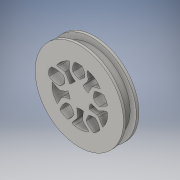
# Autodesk Inventor part: Desgin on wheel
Saved by Autodesk Inventor 2016 (Build 200138000, 138)
## iProperties
Created: 2017-09-08
Part Number: Desgin on wheel
Material: Generic
Document SubType Name: Modeling
Designer: student
Density: 1 g/cm^3
Appearance: Default
Author: student
Autodesk Inventor part; units mm, degrees
ref_plane "YZ Plane" through (0, 0, 0) normal (1, 0, 0) x (0, 1, 0)
ref_plane "XZ Plane" through (0, 0, 0) normal (0, 1, 0) x (-1, 0, 0)
ref_plane "XY Plane" through (0, 0, 0) normal (0, 0, 1) x (1, 0, 0)
sketch "Sketch1" plane through (0, 0, 0) normal (0, 0, 1) x (1, 0, 0)
  circle A0 centre (0, 0) radius 4.826
  dimension "d0" = 9.652
  constraints: 1 centre point, 1 coincident
  measures "d0" diameter of A0
extrude "Extrusion1" add sketch "Sketch1" along normal blind 3.048
sketch "Sketch2" plane through (0, 0, 3.048) normal (0, 0, 1) x (1, 0, 0)
  circle A0 centre (0, 0) radius 22.86
  dimension "d3" = 45.72
  constraints: 1 centre point, 1 coincident
  measures "d3" diameter of A0
extrude "Extrusion2" add sketch "Sketch2" along normal blind 1.397
sketch "Sketch4" plane through (0, 0, 4.445) normal (0, 0, 1) x (1, 0, 0)
  circle A0 centre (0, 0) radius 19.685
  dimension "d6" = 39.37
  constraints: 1 centre point, 1 coincident
  measures "d6" diameter of A0
extrude "Extrusion3" add sketch "Sketch4" along normal blind 5.334
sketch "Sketch6" plane through (0, 0, 9.779) normal (0, 0, 1) x (1, 0, 0)
  circle A0 centre (0, 0) radius 4.826 projected
  circle A1 centre (0, 0) radius 22.86
  constraints: 1 centre point, 1 coincident
extrude "Extrusion4" add sketch "Sketch6" along normal blind 1.27 contours A0 | A1
sketch "Sketch9" plane through (0, 0, 0) normal (0, 0, -1) x (-1, 0, 0)
  line L0 (2.3876, -2.514) -> (2.3876, 2.514)
  line L1 (-2.3876, 2.514) -> (-2.3876, -2.514)
  line L2 (-1.2735, -3.2247) -> (1.2735, 3.2247) construction
  line L3 (1.2735, -3.2247) -> (-1.2735, 3.2247) construction
  arc A0 (-2.3876, -2.514) -> (2.3876, -2.514) centre (0, 0) ccw
  arc A1 (2.3876, 2.514) -> (-2.3876, 2.514) centre (0, 0) ccw
  constraints: 8 end point, 8 point on circle, 2 centre point, 2 midpoint, 1 coincident, 1 parallel
extrude "Extrusion6" cut sketch "Sketch9" against normal blind 5.5118
sketch "Sketch10" plane through (0, 0, 3.048) normal (0, 0, -1) x (-1, 0, 0)
  arc A0 (6.0888, 12.8089) -> (4.9517, 12.8553) centre (5.4971, 12.2636) ccw
  arc A1 (11.5392, 8.311) -> (6.0888, 12.8089) centre (0.4834, 0.4651) ccw
  arc A2 (11.0546, 7.7734) -> (11.5392, 8.311) centre (11.2368, 8.0964) ccw
  arc A3 (11.0546, 7.7734) -> (7.4347, 7.1004) centre (11.1442, -2.7813) ccw
  circle A4 centre (0, 0) radius 22.86 projected
  arc A5 (5.2433, 9.0758) -> (4.9517, 12.8553) centre (-169.1009, -2.4734) ccw
  arc A6 (2.0036, 5.6242) -> (5.2433, 9.0758) centre (-1.766, 12.4088) ccw
  arc A7 (2.0036, 5.6242) -> (4.9517, 3.0409) centre (11.897, 13.941) ccw
  arc A8 (7.4347, 7.1004) -> (4.9517, 3.0409) centre (16.2062, -1.0536) ccw
  arc A9 (11.2368, -8.9724) -> (14.0004, -0.5744) centre (4.7112, -2.1713) ccw
  arc A10 (9.1497, -5.1175) -> (11.2368, -8.9724) centre (208.9836, 100.5866) ccw
  arc A11 (9.1497, -5.1175) -> (4.7112, -3.7562) centre (4.4946, -12.3784) ccw
  arc A12 (5.8832, -0.5744) -> (4.7112, -3.7562) centre (18.9185, -7.1827) ccw
  arc A13 (5.8832, -0.5744) -> (9.9506, -2.3296) centre (12.8849, 10.061) ccw
  arc A14 (9.9506, -2.3296) -> (14.0004, -0.5744) centre (5.7085, 13.0084) ccw
  arc A15 (9.9506, -11.266) -> (7.84, -7.1827) centre (1.8046, -12.8894) ccw
  arc A16 (7.84, -7.1827) -> (6.2065, -6.2202) centre (5.7633, -8.8398) ccw
  arc A17 (6.2065, -6.2202) -> (4.6733, -6.4168) centre (5.7633, -8.8398) ccw
  arc A18 (4.6733, -6.4168) -> (2.7073, -9.6817) centre (7.7197, -10.4756) ccw
  arc A19 (2.7073, -9.6817) -> (5.9896, -13.3063) centre (11.6592, -4.8738) ccw
  arc A20 (5.9896, -13.3063) -> (9.9506, -11.266) centre (2.5555, -1.7743) ccw
  arc A21 (1.2488, -5.7954) -> (-2.1893, -5.6065) centre (-0.8542, -12.6863) ccw
  arc A22 (1.2488, -5.7954) -> (0.9545, -10.3074) centre (53.2412, -11.4518) ccw
  arc A23 (3.6527, -13.5111) -> (0.9545, -10.3074) centre (-39.0545, -46.7416) ccw
  arc A24 (2.5555, -14.4106) -> (3.6527, -13.5111) centre (2.8151, -13.6083) ccw
  arc A25 (-4.8162, -13.6083) -> (2.5555, -14.4106) centre (0.014, -3.4952) ccw
  arc A26 (-4.6201, -12.8894) -> (-4.8162, -13.6083) centre (-4.1772, -13.3965) ccw
  arc A27 (-4.6201, -12.8894) -> (-1.9227, -10.3074) centre (-21.7976, 7.7557) ccw
  arc A28 (-1.9227, -10.3074) -> (-2.1893, -5.6065) centre (-14.7824, -8.6787) ccw
  arc A29 (-7.4482, -12.7759) -> (-3.5507, -9.27) centre (-12.4495, -3.2965) ccw
  arc A30 (-3.5507, -9.27) -> (-4.8162, -6.2202) centre (-13.041, -11.4205) ccw
  arc A31 (-4.8162, -6.2202) -> (-5.2818, -5.9098) centre (-5.2043, -6.2979) ccw
  arc A32 (-5.2818, -5.9098) -> (-8.2329, -5.6065) centre (-7.9223, -17.09) ccw
  arc A33 (-8.2329, -5.6065) -> (-10.6197, -10.0458) centre (-4.1164, -10.6809) ccw
  arc A34 (-10.6197, -10.0458) -> (-7.4482, -12.7759) centre (-2.1705, -3.4378) ccw
  arc A35 (2.3346, 14.0815) -> (-1.3832, 14.2076) centre (0.0752, 2.3347) ccw
  arc A36 (3.3497, 9.1954) -> (2.3346, 14.0815) centre (-2.4317, 10.5428) ccw
  arc A37 (0.5801, 7.6979) -> (3.3497, 9.1954) centre (-3.4245, 18.4144) ccw
  arc A38 (-2.849, 9.7313) -> (-0.2799, 7.7734) centre (3.746, 15.7205) ccw
  arc A39 (-1.3832, 14.2076) -> (-2.849, 9.7313) centre (3.0799, 10.268) ccw
  arc A40 (-4.6201, 3.8276) -> (-1.9227, 5.7208) centre (-7.3541, 10.5911) ccw
  arc A41 (-4.6201, 3.8276) -> (-6.7475, 7.596) centre (-37.5112, -12.2565) ccw
  arc A42 (-1.9227, 5.7208) -> (-4.3382, 8.6929) centre (-18.3879, -5.1934) ccw
  arc A43 (-4.3382, 8.6929) -> (-4.6201, 9.8732) centre (-8.7751, 8.2571) ccw
  arc A44 (-4.6201, 9.8732) -> (-4.1164, 13.3822) centre (-15.2899, 13.1953) ccw
  arc A45 (-4.1164, 13.3822) -> (-4.9848, 13.3822) centre (-4.5506, 13.1456) ccw
  arc A46 (-4.9848, 13.3822) -> (-10.7538, 8.6929) centre (-3.2343, 5.3353) ccw
  arc A47 (-6.7475, 7.596) -> (-10.7538, 8.6929) centre (-12.3706, -5.0773) ccw
  arc A48 (-7.9223, 6.0993) -> (-12.7557, 6.7633) centre (-11.4073, -1.3439) ccw
  arc A49 (-7.3541, 2.6988) -> (-7.9223, 6.0993) centre (-14.7929, 3.2035) ccw
  arc A50 (-10.4577, 0.4986) -> (-7.3541, 2.6988) centre (-11.2012, 4.8363) ccw
  arc A51 (-14.5898, 3.0409) -> (-10.4577, 0.4986) centre (-7.2589, 10.3268) ccw
  arc A52 (-12.7557, 6.7633) -> (-14.5898, 3.0409) centre (-5.9799, 1.1117) ccw
  arc A53 (-5.2818, -3.2965) -> (-6.0542, -0.2883) centre (-8.5618, -2.5354) ccw
  arc A54 (-6.0542, -0.2883) -> (-10.0183, -1.5931) centre (9.876, -55.3624) ccw
  arc A55 (-5.2818, -3.2965) -> (-9.1684, -3.8787) centre (-5.1947, -17.1417) ccw
  arc A56 (-9.1684, -3.8787) -> (-10.0183, -4.397) centre (-8.8628, -5.3359) ccw
  arc A57 (-10.0183, -1.5931) -> (-13.8141, 0.2266) centre (-38.6644, -56.4801) ccw
  arc A58 (-13.8141, 0.2266) -> (-14.5898, -0.2883) centre (-13.7445, -0.72) ccw
  arc A59 (-14.5898, -0.2883) -> (-12.122, -7.8577) centre (-4.7204, -1.2577) ccw
  arc A60 (-12.122, -7.8577) -> (-10.0183, -4.397) centre (-273.7033, 153.5242) ccw
  arc A61 (-0.2799, 7.7734) -> (0.5801, 7.6979) centre (0.2215, 8.5495) ccw
  arc A62 (8.3209, 5.3046) -> (7.4347, 2.3347) centre (11.6708, 2.6878) ccw
  arc A63 (7.4347, 2.3347) -> (10.2097, -0.443) centre (11.8697, 3.9904) ccw
  arc A64 (14.3339, 6.0011) -> (8.3209, 5.3046) centre (12.587, -5.2209) ccw
  arc A65 (15.6088, 1.087) -> (14.3339, 6.0011) centre (11.6708, 2.6878) ccw
  arc A66 (10.2097, -0.443) -> (15.6088, 1.087) centre (10.9403, 7.27) ccw
  constraints: 145 point on circle, 66 centre point, 1 concentric, 1 tangent
extrude "Extrusion7" cut sketch "Sketch10" against normal through all contours A1 A2 A3 A8 A7 A6 A5 A0 | A10 A11 A12 A13 A14 A9 | A20 A19 A18 A17 A16 A15 | A22 A23 A24 A25 A26 A27 A28 A21 | A34 A33 A32 A31 A30 A29 | A36 A37 A61 A38 A39 A35 | A41 A47 A46 A45 A44 A43 A42 A40 | A49 A50 A51 A52 A48 | A55 A56 A60 A59 A58 A57 A54 A53 | A64 A65 A66 A63 A62
body "Solid1"
